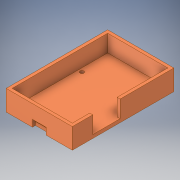
# Autodesk Inventor part: Raspi3B+_Case
Saved by Autodesk Inventor 2018 (Build 220112000, 112)
## iProperties
Created: 2018-06-22
Part Number: Raspi3B+_Case
Material: Generic
Document SubType Name: Modeling
Designer: snipe
Density: 1 g/cm^3
Appearance: Default
Sending System: SolidWorks 2017
Last Author: Dan
Last Saved: 2018-12-13
Author: snipe
Autodesk Inventor part; units mm, degrees
ref_plane "YZ Plane" through (0, 0, 0) normal (1, 0, 0) x (0, 1, 0)
ref_plane "XZ Plane" through (0, 0, 0) normal (0, 1, 0) x (-1, 0, 0)
ref_plane "XY Plane" through (0, 0, 0) normal (0, 0, 1) x (1, 0, 0)
ref_plane "Work Plane3" through (-25, 0, 42.5) normal (0, -1, 0) x (1, 0, 0)
sketch "Sketch1" plane through (-25, 0, 42.5) normal (0, -1, 0) x (1, 0, 0)
  line L0 (28.4781, -19.558) -> (28.4781, -33.5534) projected
  arc A0 (53, -3) -> (50, 0) centre (50, -3) ccw projected
  line L1 (0, 0) -> (50, 0) projected
  arc A1 (0, 0) -> (-3, -3) centre (0, -3) ccw projected
  line L2 (-3, -82) -> (-3, -3) projected
  arc A2 (-3, -82) -> (0, -85) centre (0, -82) ccw projected
  line L3 (50, -85) -> (0, -85) projected
  arc A3 (50, -85) -> (53, -82) centre (50, -82) ccw projected
  line L4 (53, -3) -> (53, -82) projected
  circle A4 centre (49.5, -61.5) radius 1.75 projected
  circle A5 centre (0.5, -61.5) radius 1.75 projected
  circle A6 centre (0.5, -3.5) radius 1.75 projected
  circle A7 centre (49.5, -3.5) radius 1.75 projected
  line L5 (-3, 0) -> (53, 0)
  line L6 (53, 0) -> (53, -88.9)
  line L7 (53, -88.9) -> (-3, -88.9)
  line L8 (-3, -88.9) -> (-3, 0)
  point P0 (25, -42.5)
  dimension "d0" = 88.9
  constraints: 8 end point, 2 parallel, 1 horizontal, 1 perpendicular, 1 point on line
  measures "d0" distance of L5.end L6.end
extrude "Extrusion1" add sketch "Sketch1" along normal blind 3.175
sketch "Sketch2" plane through (-25, -3.175, 42.5) normal (0, -1, 0) x (1, 0, 0)
  circle A0 centre (49.5, -3.5) radius 1.75 projected
  circle A1 centre (0.5, -3.5) radius 1.75 projected
  circle A2 centre (0.5, -61.5) radius 1.75 projected
  circle A3 centre (49.5, -61.5) radius 1.75 projected
  line L0 (53, 0) -> (-3, 0) projected
  line L1 (-3, 0) -> (-3, -88.9) projected
  line L2 (-3, -88.9) -> (53, -88.9) projected
  line L3 (53, -88.9) -> (53, 0) projected
  line L4 (-3, -88.9) -> (53, -88.9) projected
  line L5 (55.8, 2.8) -> (55.8, -91.7)
  line L6 (-5.8, -91.7) -> (-5.8, 2.8)
  line L7 (53, 0) -> (55.8, 2.8)
  line L8 (53, 0) -> (58.3967, 0) construction
  line L9 (55.8, 2.8) -> (-5.8, 2.8)
  line L10 (53, -88.9) -> (61.5609, -88.9) construction
  line L11 (55.8, -91.7) -> (-5.8, -91.7)
  point P0 (25, -42.5)
  dimension "d3" = 45
  constraints: 14 end point, 4 horizontal, 1 parallel
  measures "d3" angle of L8 L7
extrude "Extrusion2" add sketch "Sketch2" against normal blind 19.05 contours L5 L11 L6 L9
sketch "Sketch3" plane through (-25, 15.875, 42.5) normal (0, 1, 0) x (1, 0, 0)
  line L0 (-3, 0) -> (-3, 88.9) projected
  line L1 (-3, 88.9) -> (53, 88.9) projected
  line L2 (53, 88.9) -> (53, 0) projected
  line L3 (53, 0) -> (-3, 0) projected
  line L4 (-5.8, -2.8) -> (55.8, -2.8) projected
  line L5 (55.8, -2.8) -> (55.8, 91.7) projected
  line L6 (55.8, 91.7) -> (-5.8, 91.7) projected
  line L7 (-5.8, 91.7) -> (-5.8, -2.8) projected
  line L8 (53, 16.25) -> (55.8, 16.25)
  line L9 (55.8, 16.25) -> (55.8, 41.65)
  line L10 (55.8, 41.65) -> (53, 41.65)
  line L11 (53, 41.65) -> (53, 16.25)
  point P0 (25, 42.5)
  dimension "d7" = 19.05
  dimension "d8" = 25.4
  constraints: 8 end point, 2 parallel, 2 point on line, 1 horizontal, 1 perpendicular
  measures "d7" distance between parallel lines of L4 L8
  measures "d8" distance between parallel lines of L10 L8
extrude "Extrusion3" cut sketch "Sketch3" against normal blind 15.875 contours L2 L10 L5 L8
sketch "Sketch4" plane through (-25, -3.175, 42.5) normal (0, -1, 0) x (1, 0, 0)
  line L0 (55.8, 2.8) -> (-5.8, 2.8) projected
  line L1 (18.65, -0.0575) -> (31.35, -0.0575)
  line L2 (31.35, -0.0575) -> (31.35, 2.8)
  line L3 (31.35, 2.8) -> (18.65, 2.8)
  line L4 (18.65, 2.8) -> (18.65, -0.0575)
  line L5 (25, 21.7) -> (25, -110.6) projected
  point P0 (25, -42.5)
  dimension "d11" = 12.7
  dimension "d12" = 2.8575
  constraints: 8 end point, 2 parallel, 1 horizontal, 1 perpendicular, 1 point on line, 1 other
  measures "d11" distance between parallel lines of L2 L4
  measures "d12" distance between parallel lines of L0 L1
extrude "Extrusion4" cut sketch "Sketch4" against normal blind 6.35
body "Solid1"
